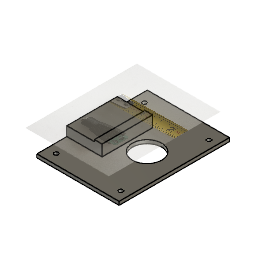
charing_dock_back (Autodesk Fusion 360 design; units mm, degrees)
part number: 2026-07-18-17-42-37-291
Autodesk Fusion 360 part; units mm, degrees
sketch "Sketch1" plane through (0, 0, 0) normal (0, 0, 1) x (1, 0, 0)
  line L0 (0, 0) -> (70, 0)
  line L1 (70, 0) -> (70, 54)
  line L2 (70, 54) -> (0, 54)
  line L3 (0, 54) -> (0, 0)
  line L4 (0, 0) -> (70, 0)
  line L5 (70, 0) -> (70, -20)
  line L6 (70, -20) -> (0, -20)
  line L7 (0, -20) -> (0, 0)
  line L8 (0, 54) -> (70, 54)
  line L9 (70, 54) -> (70, 74)
  line L10 (70, 74) -> (0, 74)
  line L11 (0, 74) -> (0, 54)
  dimension "d1" = 54
  dimension "d2" = 70
  dimension "d3" = 20
  dimension "d4" = 20
  constraint horizontal L0
  constraint vertical L1
  constraint horizontal L2
  constraint vertical L3
  constraint coincident L0.start L3.end
  constraint horizontal L4
  constraint vertical L5
  constraint horizontal L6
  constraint vertical L7
  constraint horizontal L8
  constraint vertical L9
  constraint horizontal L10
  constraint vertical L11
  measures "d1" distance of L0.start L2.end
  measures "d2" distance of L0.start L0.end
  measures "d3" distance of L0.start L6.end
  measures "d4" distance of L2.end L10.end
extrude "Extrude1" add sketch "Sketch1" along normal blind 3
hole "Hole1" at (45.2511, 28.5377, 3) direction (0, 0, -1) diameter 25 depth 5 tip angle 180
sketch "Sketch3" plane through (0, 0, 3) normal (0, 0, 1) x (-1, 0, 0)
  circle A0 centre (-45.2511, -28.5377) radius 12.5
  line L0 (0, -48.5) -> (-30.0019, -48.5)
  line L1 (-30.0019, -48.5) -> (-30.0019, -5.5)
  line L2 (-30.0019, -5.5) -> (0, -5.5)
  line L3 (0, -5.5) -> (0, -48.5)
  line L4 (-70, 20) -> (-70, -74)
  line L5 (-70, -74) -> (0, -74)
  line L6 (0, -74) -> (0, 20)
  line L7 (0, 20) -> (-70, 20)
  dimension "d20" = 25.5
  dimension "d21" = 25.5
  constraint horizontal L0
  constraint vertical L1
  constraint horizontal L2
  constraint vertical L3
  constraint collinear L3 L6
  measures "d20" distance of L2 L7
  measures "d21" distance of L0 L5
extrude "Extrude3" add sketch "Sketch3" along normal blind 8 contours L0 L1 L2 L3 L6
sketch "Sketch4" plane through (0, 0, 3) normal (0, 0, 1) x (-1, 0, 0)
  line L0 (0, -48.5) -> (-30.0019, -48.5)
  line L1 (-30.0019, -48.5) -> (-30.0019, -5.5)
  line L2 (-30.0019, -5.5) -> (0, -5.5)
  line L3 (0, -5.5) -> (0, 20)
  line L4 (0, 20) -> (-70, 20)
  line L5 (-70, 20) -> (-70, -74)
  line L6 (-70, -74) -> (0, -74)
  line L7 (0, -74) -> (0, -48.5)
  circle A0 centre (-45.2511, -28.5377) radius 12.5
  circle A1 centre (-8, -63.531) radius 1.75
  circle A2 centre (-63, -63.531) radius 1.75
  circle A3 centre (-8, 11.469) radius 1.75
  circle A4 centre (-63, 11.469) radius 1.75
  dimension "d22" = 3.5
  dimension "d25" = -55
  dimension "d26" = 75
  dimension "d27" = 10.469
  dimension "d30" = 8
  measures "d22" diameter of A1
  measures "d27" distance of L6 A1.centre
  measures "d30" distance of L7 A1.centre
extrude "Extrude4" cut sketch "Sketch4" against normal blind 3 contours A1 | A2 | A3 | A4
sketch "Sketch5" plane through (0, 0, 11) normal (0, 0, 1) x (-1, 0, 0)
  line L0 (0, -5.5) -> (-30.0019, -5.5)
  line L1 (-30.0019, -5.5) -> (-30.0019, -48.5)
  line L2 (-30.0019, -48.5) -> (0, -48.5)
  line L3 (0, -48.5) -> (0, -5.5)
  line L4 (-30.0019, -5.5) -> (-23.4899, -5.5)
  line L5 (-23.4899, -5.5) -> (-23.4899, -48.5)
  line L6 (-23.4899, -48.5) -> (-30.0019, -48.5)
  line L7 (-30.0019, -48.5) -> (-30.0019, -5.5)
  constraint horizontal L4
  constraint vertical L5
  constraint horizontal L6
  constraint vertical L7
  constraint coincident L2 L5.end
  constraint coincident L0.end L1.start
extrude "Extrude5" add sketch "Sketch5" along normal blind 1.5 contours L0 L1 L2 L4 L5 L6 L7
